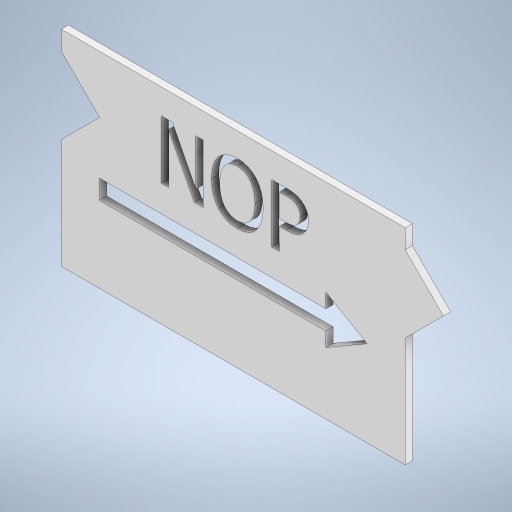
# Autodesk Inventor part: MS_R_Front_top_yellow_v3
Saved by Autodesk Inventor 2024 (Build 280153000, 153)
## iProperties
Created: 2024-02-15
Part Number: MS_R_Front_top_yellow_v3
Material: Generic
Document SubType Name: Modeling
Designer: LKLM
Density: 1 g/cm^3
Appearance: White
Author: LKLM
Autodesk Inventor part; units mm, degrees
ref_plane "YZ Plane" through (0, 0, 0) normal (1, 0, 0) x (0, 1, 0)
ref_plane "XZ Plane" through (0, 0, 0) normal (0, 1, 0) x (-1, 0, 0)
ref_plane "XY Plane" through (0, 0, 0) normal (0, 0, 1) x (1, 0, 0)
sketch "Sketch1" plane through (0, 0, 0) normal (0, 0, 1) x (1, 0, 0)
  circle A0 centre (-72, 68) radius 8 construction
  line L0 (-72, 60) -> (0, 60) construction
  line L1 (-72, 76) -> (-64, 68)
  line L2 (-72, 60) -> (-64, 68)
  line L3 (-72, 76) -> (-72, 80)
  line L4 (0, 76) -> (0, 80)
  line L5 (-72, 80) -> (0, 80)
  line L6 (-72, 76) -> (11.4847, 76) construction
  line L7 (-64, 68) -> (11.3495, 68) construction
  line L8 (-72, 60) -> (23.0654, 60) construction
  circle A1 centre (0, 68) radius 8 construction
  line L9 (0, 60) -> (8, 68)
  line L10 (8, 68) -> (0, 76)
  line L11 (-34, 51.1) -> (-34, 39.9508) construction
  line L12 (-36, 51.1) -> (-36, 38.5) construction
  line L13 (0, 37) -> (-91.064, 37) construction
  line L14 (0, 37) -> (-72, 37)
  line L15 (-64, 68) -> (-64, -7.5721) construction
  line L16 (31.0795, 0) -> (31.0795, 55) construction
  line L17 (31.0795, 55) -> (-111.8136, 55) construction
  line L18 (-8, 68) -> (-8, -20.4909) construction
  line L19 (-8, 55) -> (-16.6, 55) construction
  line L20 (-16.6, 55) -> (-16.6, 50) construction
  line L21 (-16.6, 50) -> (-8, 55)
  line L22 (-16.6, 60) -> (-8, 55)
  line L23 (-16.6, 50) -> (-16.6, 53)
  line L24 (-16.6, 53) -> (-64, 53)
  line L25 (-64, 53) -> (-64, 57)
  line L26 (-64, 57) -> (-16.6, 57)
  line L27 (-16.6, 57) -> (-16.6, 60)
  line L28 (-72, 37) -> (-72, 60)
  line L29 (-72, 35.1512) -> (-72, 37)
  line L30 (0, 60) -> (0, 37)
  point P0 (0, 78)
  point P1 (-72, 78)
  point P2 (-137.4598, 47.0487)
  dimension "d5" = 72
  dimension "d50" = 55
  dimension "d51" = 8.6
  dimension "d52" = 5
  dimension "d54" = 4
  dimension "d55" = 1.5
  constraints: 62 end point, 14 point on line, 6 perpendicular, 6 point on circle, 5 tangent, 4 parallel, 3 horizontal, 3 vertical, 2 centre point, 2 collinear, 2 midpoint
  measures "d5" distance of point (0, 78) point (-72, 78)
  measures "d50" distance of L16.start L16.end
  measures "d51" distance of L19.start L19.end
  measures "d52" distance of L19.end L20.end
  measures "d54" distance of L24.end L25.end
  measures "d55" distance from line of L14 L12.end
extrude "Extrusion7" add sketch "Sketch1" along normal blind 1.5
sketch "Sketch10" plane through (0, 0, 1.5) normal (0, 0, 1) x (1, 0, 0)
  line L0 (-52.276, 75.0151) -> (-43.77, 75.0151) construction
  line L1 (-43.77, 75.0151) -> (-43.77, 65.3644) construction
  line L2 (-43.77, 65.3644) -> (-52.276, 65.3644) construction
  line L3 (-52.276, 65.3644) -> (-52.276, 75.0151) construction
  line L4 (-42.3103, 62.5581) -> (-44.1294, 62.5581)
  line L5 (-44.1294, 62.5581) -> (-49.5275, 73.0774)
  line L6 (-49.5275, 73.0774) -> (-49.5275, 62.5581)
  line L7 (-49.5275, 62.5581) -> (-51.0401, 62.5581)
  line L8 (-51.0401, 62.5581) -> (-51.0401, 74.7581)
  line L9 (-51.0401, 74.7581) -> (-48.7366, 74.7581)
  line L10 (-48.7366, 74.7581) -> (-43.823, 65.0989)
  line L11 (-43.823, 65.0989) -> (-43.823, 74.7581)
  line L12 (-43.823, 74.7581) -> (-42.3103, 74.7581)
  line L13 (-42.3103, 74.7581) -> (-42.3103, 62.5581)
  spline S0 degree 2 poles (-31.2077, 73.3641) (-30.5157, 72.5534) (-29.7445, 70.1806) (-29.7445, 68.6581) knots 0 0 0 1 2 2 2
  spline S1 degree 2 poles (-29.7445, 68.6581) (-29.7445, 67.1751) (-30.4959, 64.7727) (-31.2077, 63.962) knots 0 0 0 1 2 2 2
  spline S2 degree 2 poles (-31.2077, 63.962) (-31.9591, 63.1117) (-33.9463, 62.301) (-35.1426, 62.301) knots 0 0 0 1 2 2 2
  spline S3 degree 2 poles (-35.1426, 62.301) (-36.3784, 62.301) (-38.3557, 63.1414) (-39.0774, 63.962) knots 0 0 0 1 2 2 2
  spline S4 degree 2 poles (-39.0774, 63.962) (-39.7794, 64.7727) (-40.5307, 67.1553) (-40.5307, 68.6581) knots 0 0 0 1 2 2 2
  spline S5 degree 2 poles (-40.5307, 68.6581) (-40.5307, 70.1905) (-39.7695, 72.5237) (-39.0675, 73.3641) knots 0 0 0 1 2 2 2
  spline S6 degree 2 poles (-39.0675, 73.3641) (-38.3557, 74.1748) (-36.3685, 75.0151) (-35.1426, 75.0151) knots 0 0 0 1 2 2 2
  spline S7 degree 2 poles (-35.1426, 75.0151) (-33.8969, 75.0151) (-31.8998, 74.1451) (-31.2077, 73.3641) knots 0 0 0 1 2 2 2
  spline S8 degree 2 poles (-31.4351, 68.6581) (-31.4351, 69.8642) (-31.9591, 71.7328) (-32.4337, 72.3458) knots 0 0 0 1 2 2 2
  spline S9 degree 2 poles (-32.4337, 72.3458) (-32.9181, 72.9785) (-34.2824, 73.6112) (-35.1327, 73.6112) knots 0 0 0 1 2 2 2
  spline S10 degree 2 poles (-35.1327, 73.6112) (-36.0126, 73.6112) (-37.3374, 72.9983) (-37.8416, 72.3458) knots 0 0 0 1 2 2 2
  spline S11 degree 2 poles (-37.8416, 72.3458) (-38.326, 71.7229) (-38.8401, 69.8445) (-38.8401, 68.6581) knots 0 0 0 1 2 2 2
  spline S12 degree 2 poles (-38.8401, 68.6581) (-38.8401, 66.2556) (-36.8233, 63.7049) (-35.1327, 63.7049) knots 0 0 0 1 2 2 2
  spline S13 degree 2 poles (-35.1327, 63.7049) (-33.4421, 63.7049) (-31.4351, 66.2556) (-31.4351, 68.6581) knots 0 0 0 1 2 2 2
  spline S14 degree 2 poles (-20.2534, 71.0803) (-20.2534, 70.2894) (-20.817, 68.8657) (-21.3212, 68.3714) knots 0 0 0 1 2 2 2
  spline S15 degree 2 poles (-21.3212, 68.3714) (-21.9539, 67.7485) (-23.6643, 67.1059) (-24.9693, 67.1059) knots 0 0 0 1 2 2 2
  line L14 (-24.9693, 67.1059) -> (-26.3435, 67.1059)
  line L15 (-26.3435, 67.1059) -> (-26.3435, 62.5581)
  line L16 (-26.3435, 62.5581) -> (-27.9649, 62.5581)
  line L17 (-27.9649, 62.5581) -> (-27.9649, 74.7581)
  line L18 (-27.9649, 74.7581) -> (-24.9001, 74.7581)
  spline S16 degree 2 poles (-24.9001, 74.7581) (-23.8126, 74.7581) (-22.2901, 74.4022) (-21.7068, 73.9968) knots 0 0 0 1 2 2 2
  spline S17 degree 2 poles (-21.7068, 73.9968) (-21.0246, 73.5321) (-20.2534, 72.0986) (-20.2534, 71.0803) knots 0 0 0 1 2 2 2
  spline S18 degree 2 poles (-21.944, 71.0308) (-21.944, 71.6636) (-22.379, 72.5929) (-22.8239, 72.8895) knots 0 0 0 1 2 2 2
  spline S19 degree 2 poles (-22.8239, 72.8895) (-23.2095, 73.1466) (-24.2377, 73.3542) (-24.999, 73.3542) knots 0 0 0 1 2 2 2
  line L19 (-24.999, 73.3542) -> (-26.3435, 73.3542)
  line L20 (-26.3435, 73.3542) -> (-26.3435, 68.49)
  line L21 (-26.3435, 68.49) -> (-25.2363, 68.49)
  spline S20 degree 2 poles (-25.2363, 68.49) (-24.2476, 68.49) (-23.0316, 68.8064) (-22.6361, 69.2216) knots 0 0 0 1 2 2 2
  spline S21 degree 2 poles (-22.6361, 69.2216) (-22.2703, 69.5874) (-21.944, 70.4475) (-21.944, 71.0308) knots 0 0 0 1 2 2 2
  point P0 (0, 0)
  constraints: 2 other
extrude "Extrusion11" cut sketch "Sketch10" against normal up to surface (1.5 mm away)
body "Solid4"
